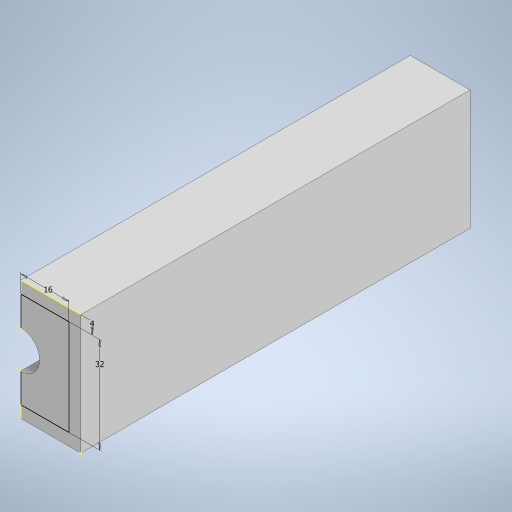
# Autodesk Inventor part: hard_support_wm
Saved by Autodesk Inventor 2023 (Build 270158000, 158)
## iProperties
Created: 2024-07-25
Part Number: hard_support_wm
Material: 일반
Document SubType Name: Modeling
Designer: ojs08
Density: 1 g/cm^3
Appearance: 기본값
Author: ojs08
Autodesk Inventor part; units mm, degrees
ref_plane "YZ Plane" through (0, 0, 0) normal (1, 0, 0) x (0, 1, 0)
ref_plane "XZ Plane" through (0, 0, 0) normal (0, 1, 0) x (-1, 0, 0)
ref_plane "XY Plane" through (0, 0, 0) normal (0, 0, 1) x (1, 0, 0)
sketch "스케치1" plane through (0, 0, 0) normal (0, 0, 1) x (1, 0, 0)
  line L0 (0, 0) -> (-20, 0)
  line L1 (-20, 0) -> (-20, 40)
  line L2 (-20, 40) -> (0, 40)
  line L3 (0, 40) -> (0, 0)
  circle A0 centre (-20, 20) radius 6.25
  point P0 (-20, 26.25)
  point P1 (-20, 13.75)
  dimension "d0" = 40
  dimension "d1" = 20
  dimension "d2" = 20
  dimension "d3" = 12.5
  constraints: 8 end point, 2 parallel, 1 centre point, 1 coincident, 1 horizontal, 1 midpoint, 1 perpendicular
  measures "d0" distance of L2.end L0.start
  measures "d1" distance of L0.start L0.end
  measures "d2" distance of L1.end A0.centre
  measures "d3" diameter of A0
extrude "돌출1" add sketch "스케치1" along normal blind 130 contours L0 L1 A0 L2 L3
sketch "스케치2" plane through (0, 0, 130) normal (0, 0, 1) x (1, 0, 0)
  line L0 (-20, 40) -> (-20, 26.25) projected
  line L1 (-20, 36) -> (-4, 36)
  line L2 (-4, 36) -> (-4, 4)
  line L3 (-4, 4) -> (-20, 4)
  line L4 (-20, 13.75) -> (-20, 0) projected
  line L5 (0, 40) -> (-20, 40) projected
  point P0 (0, 0)
  dimension "d6" = 16
  dimension "d7" = 32
  dimension "d8" = 4
  constraints: 6 end point, 2 perpendicular, 1 horizontal, 1 point on line
  measures "d6" distance of L1.start L1.end
  measures "d7" distance of L1.end L2.end
  measures "d8" distance between parallel lines of L5 L1
sketch "스케치3" plane through (0, 0, 130) normal (0, 0, 1) x (1, 0, 0)
  line L0 (-20, 36) -> (-4, 36) projected
  line L1 (-4, 36) -> (-4, 4) projected
  line L2 (-4, 4) -> (-20, 4) projected
  line L3 (-20, 13.75) -> (-20, 0) projected
  line L4 (-20, 40) -> (-20, 26.25) projected
  point P0 (0, 0)
sketch "스케치4" plane through (0, 0, 130) normal (0, 0, 1) x (1, 0, 0)
  line L0 (-20, 40) -> (-20, 26.25) projected
  line L1 (-20, 35.8924) -> (-20, 26.25)
  line L2 (-20, 13.75) -> (-20, 0) projected
  line L3 (-20, 4.1853) -> (-20, 13.75)
  point P0 (0, 0)
  constraints: 4 end point, 2 collinear, 1 point on line
sketch "스케치5" plane through (0, 0, 130) normal (0, 0, 1) x (1, 0, 0)
  line L0 (-20, 36) -> (-4, 36) projected
  line L1 (-4, 36) -> (-4, 4) projected
  line L2 (-4, 4) -> (-20, 4) projected
  line L3 (-20, 13.75) -> (-20, 0) projected
  line L4 (-20, 40) -> (-20, 26.25) projected
  point P0 (0, 0)
  point P1 (-20, 4.1853)
sketch "스케치6" plane through (0, 0, 0) normal (0, 0, -1) x (-1, 0, 0)
  line L0 (20, 13.75) -> (20, 0) projected
  line L1 (20, 4) -> (4, 4)
  line L2 (4, 4) -> (4, 36)
  line L3 (4, 36) -> (20, 36)
  line L4 (20, 36) -> (20, 4)
  line L5 (20, 0) -> (0, 0) projected
  arc A0 (20, 26.25) -> (20, 13.75) centre (20, 20) ccw projected
  dimension "d9" = 16
  dimension "d10" = 32
  dimension "d11" = 4
  constraints: 8 end point, 2 parallel, 1 horizontal, 1 perpendicular, 1 point on line
  measures "d9" distance of L1.start L1.end
  measures "d10" distance of L1.end L2.end
  measures "d11" distance between parallel lines of L5 L1
extrude "돌출2" cut sketch "스케치6" against normal blind 100 contours L0 L1 L2 L3 L4 A0
sketch "스케치7" plane through (-20, 0, 130) normal (-1, 0, 0) x (0, 0, 1)
  circle A0 centre (-15, 6.25) radius 5.4
  circle A1 centre (-15, 33.75) radius 5.4
  line L0 (0, 13.75) -> (0, 0) projected
  line L1 (-30, 13.75) -> (0, 13.75) projected
  line L2 (0, 40) -> (0, 26.25) projected
  line L3 (-130, 40) -> (0, 40) projected
  point P0 (-130, 0)
  dimension "d14" = 10.8
  dimension "d15" = 10.8
  dimension "d16" = 15
  dimension "d17" = 7.5
  dimension "d18" = 15
  dimension "d19" = 6.25
  constraints: 2 centre point
  measures "d14" diameter of A0
  measures "d15" diameter of A1
  measures "d16" distance from line of L0 A0.centre
  measures "d17" distance from line of L1 A0.centre
  measures "d18" distance from line of L2 A1.centre
  measures "d19" distance from line of L3 A1.centre
extrude "돌출3" cut sketch "스케치7" against normal blind 10.4
